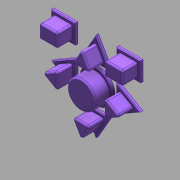
# Autodesk Inventor part: Button
Saved by Autodesk Inventor 2016 (Build 200138000, 138)
## iProperties
Created: 2016-08-15
Part Number: Button
Material: Water
Document SubType Name: Modeling
Designer: ADMIN
Density: 0.9983 g/cm^3
Appearance: Violet
Author: ADMIN
Autodesk Inventor part; units mm, degrees
ref_plane "YZ Plane" through (0, 0, 0) normal (1, 0, 0) x (0, 1, 0)
ref_plane "XZ Plane" through (0, 0, 0) normal (0, 1, 0) x (-1, 0, 0)
ref_plane "XY Plane" through (0, 0, 0) normal (0, 0, 1) x (1, 0, 0)
sketch "Sketch7" plane through (0, 0, 0) normal (0, 1, 0) x (-1, 0, 0)
  circle A0 centre (0, 0) radius 15
  line L0 (-25, 0) -> (-25, 10)
  line L1 (-25, 0) -> (-25, -10)
  line L2 (-25, -10) -> (-42.3205, 0)
  line L3 (-42.3205, 0) -> (-25, 10)
  line L4 (-22, 15.1962) -> (-22, 0)
  line L5 (-22, 0) -> (-22, -15.1962)
  line L6 (-22, -15.1962) -> (-48.3205, 0)
  line L7 (-48.3205, 0) -> (-22, 15.1962)
  circle A1 centre (0, 0) radius 18
  line L8 (0, -25) -> (-10, -25)
  line L9 (0, -25) -> (10, -25)
  line L10 (10, -25) -> (0, -42.3205)
  line L11 (0, -42.3205) -> (-10, -25)
  line L12 (-15.1962, -22) -> (0, -22)
  line L13 (0, -22) -> (15.1962, -22)
  line L14 (15.1962, -22) -> (0, -48.3205)
  line L15 (0, -48.3205) -> (-15.1962, -22)
  line L16 (25, 0) -> (25, -10)
  line L17 (25, 0) -> (25, 10)
  line L18 (25, 10) -> (42.3205, 0)
  line L19 (42.3205, 0) -> (25, -10)
  line L20 (22, -15.1962) -> (22, 0)
  line L21 (22, 0) -> (22, 15.1962)
  line L22 (22, 15.1962) -> (48.3205, 0)
  line L23 (48.3205, 0) -> (22, -15.1962)
  line L24 (0, 25) -> (10, 25)
  line L25 (0, 25) -> (-10, 25)
  line L26 (-10, 25) -> (0, 42.3205)
  line L27 (0, 42.3205) -> (10, 25)
  line L28 (15.1962, 22) -> (0, 22)
  line L29 (0, 22) -> (-15.1962, 22)
  line L30 (-15.1962, 22) -> (0, 48.3205)
  line L31 (0, 48.3205) -> (15.1962, 22)
  line L32 (48.3205, 48.3205) -> (22.3205, 48.3205)
  line L33 (22.3205, 48.3205) -> (22.3205, 27.3205)
  line L34 (22.3205, 27.3205) -> (48.3205, 27.3205)
  line L35 (48.3205, 27.3205) -> (48.3205, 48.3205)
  line L36 (-48.3205, 48.3205) -> (-22.3205, 48.3205)
  line L37 (-22.3205, 48.3205) -> (-22.3205, 27.3205)
  line L38 (-22.3205, 27.3205) -> (-48.3205, 27.3205)
  line L39 (-48.3205, 27.3205) -> (-48.3205, 48.3205)
  line L40 (45.3205, 45.3205) -> (25.3205, 45.3205)
  line L41 (25.3205, 45.3205) -> (25.3205, 30.3205)
  line L42 (25.3205, 30.3205) -> (45.3205, 30.3205)
  line L43 (45.3205, 30.3205) -> (45.3205, 45.3205)
  line L44 (-25.3205, 30.3205) -> (-25.3205, 45.3205)
  line L45 (-25.3205, 45.3205) -> (-45.3205, 45.3205)
  line L46 (-45.3205, 45.3205) -> (-45.3205, 30.3205)
  line L47 (-45.3205, 30.3205) -> (-25.3205, 30.3205)
  dimension "d85" = 10
  dimension "d86" = 10
  dimension "d87" = 20
  dimension "d88" = 60
  dimension "d89" = 3
  dimension "d90" = 3
  dimension "d93" = 360
  dimension "d95" = 26
  dimension "d96" = 21
  dimension "d97" = 26
  dimension "d98" = 21
  dimension "d99" = 3
  dimension "d100" = 3
  constraints: 96 end point, 8 parallel, 4 perpendicular, 2 centre point, 2 horizontal, 2 vertical, 1 coincident, 1 point on line, 74 other
  measures "d85" distance of L0.start L0.end
  measures "d86" distance of L0.start L1.end
  measures "d87" distance of L1.end L2.end
  measures "d88" angle of L1 L2
  measures "d89" distance between parallel lines of L0 L4
  measures "d90" radial gap between concentric circles of A0 A1
  measures "d95" distance of L34.end L33.end
  measures "d96" distance of L33.end L32.end
  measures "d97" distance of L37.end L38.end
  measures "d98" distance of L36.end L37.end
  measures "d99" distance between parallel lines of L35 L43
  measures "d100" distance between parallel lines of L37 L44
extrude "Extrusion3" add sketch "Sketch7" against normal blind 4
sketch "Sketch8" plane through (0, 0, 0) normal (0, 1, 0) x (1, 0, 0)
  line L0 (-25, -10) -> (-25, 10) projected
  line L1 (-25, -10) -> (-42.3205, 0) projected
  line L2 (-25, 10) -> (-42.3205, 0)
  line L3 (-42.3205, 0) -> (-25, -10)
  line L4 (-25, -10) -> (-25, 10)
  line L5 (-25.3205, -30.3205) -> (-45.3205, -30.3205) projected
  line L6 (-45.3205, -30.3205) -> (-25.3205, -30.3205)
  line L7 (-25.3205, -30.3205) -> (-25.3205, -45.3205)
  line L8 (-25.3205, -45.3205) -> (-45.3205, -45.3205)
  line L9 (-45.3205, -45.3205) -> (-45.3205, -30.3205)
  line L10 (25.3205, -30.3205) -> (45.3205, -30.3205)
  line L11 (45.3205, -30.3205) -> (45.3205, -45.3205)
  line L12 (45.3205, -45.3205) -> (25.3205, -45.3205)
  line L13 (25.3205, -45.3205) -> (25.3205, -30.3205)
  line L14 (-10, -25) -> (0, -42.3205)
  line L15 (0, -42.3205) -> (10, -25)
  line L16 (10, -25) -> (-10, -25)
  line L17 (25, -10) -> (42.3205, 0)
  line L18 (42.3205, 0) -> (25, 10)
  line L19 (25, 10) -> (25, -10)
  line L20 (10, 25) -> (0, 42.3205)
  line L21 (0, 42.3205) -> (-10, 25)
  line L22 (-10, 25) -> (10, 25)
  circle A0 centre (0, 0) radius 15
  dimension "d103" = 20
  dimension "d104" = 15
  dimension "d105" = 20
  dimension "d106" = 15
  dimension "d109" = 360
  dimension "d111" = 30
  constraints: 40 end point, 6 equal length, 2 horizontal, 2 perpendicular, 1 centre point, 1 coincident, 25 other
  measures "d103" distance of L7.end L8.end
  measures "d104" distance of L6.end L7.end
  measures "d105" distance of L11.end L12.end
  measures "d106" distance of L10.end L11.end
  measures "d111" diameter of A0
extrude "Extrusion4" add sketch "Sketch8" against normal blind 20
sketch "Sketch9" plane through (0, 0, 0) normal (0, 1, 0) x (1, 0, 0)
  circle A0 centre (-7.5, 0) radius 1.5
  circle A1 centre (0, -37) radius 1.5
  circle A2 centre (-40, -37.8205) radius 1.5
  circle A3 centre (40, -37.8205) radius 1.5
  circle A4 centre (37, 0) radius 1.5
  circle A5 centre (0, 37) radius 1.5
  circle A6 centre (-37, 0) radius 1.5
  point P0 (0, 0)
  dimension "d114" = 3
  dimension "d115" = 3
  dimension "d116" = 3
  dimension "d117" = 3
  dimension "d120" = 360
  constraints: 7 centre point, 9 other
  measures "d114" diameter of A0
  measures "d115" diameter of A1
  measures "d116" diameter of A2
  measures "d117" diameter of A3
extrude "Extrusion5" cut sketch "Sketch9" against normal blind 12
fillet "Fillet12" radius 2 21 edges at (45.3205, -12, 45.3205) (25.3205, -12, 45.3205) (25.3205, -12, 30.3205) (45.3205, -12, 30.3205) (42.3205, -12, 0) (25, -12, 10) (25, -12, -10) (0, -12, -42.3205) (-10, -12, -25) (10, -12, -25) (-42.3205, -12, 0) (-25, -12, -10) (-25, -12, 10) (-45.3205, -12, 30.3205) (-10, -12, 25) (0, -12, 42.3205) (-45.3205, -12, 45.3205) (-25.3205, -12, 45.3205) (10, -12, 25) (-25.3205, -12, 30.3205) (-15, -20, 0)
fillet "Fillet13" radius 2 40 edges at (44.7347, -20, 44.7347) (35.3205, -20, 45.3205) (25.9063, -20, 44.7347) (25.3205, -20, 37.8205) (25.9063, -20, 30.9063) (35.3205, -20, 30.3205) (44.7347, -20, 30.9063) (45.3205, -20, 37.8205) (0, -20, 40.3205) (-5, -20, 33.6603) (-8.2679, -20, 26) (0, -20, 25) (8.2679, -20, 26) (5, -20, 33.6603) (26, -20, 8.2679) (25, -20, 0) (26, -20, -8.2679) (33.6603, -20, -5) (40.3205, -20, 0) (33.6603, -20, 5) (-25.9063, -20, 44.7347) (-35.3205, -20, 45.3205) (-44.7347, -20, 44.7347) (-45.3205, -20, 37.8205) (-44.7347, -20, 30.9063) (-35.3205, -20, 30.3205) (-25.9063, -20, 30.9063) (-25.3205, -20, 37.8205) (-26, -20, 8.2679) (-33.6603, -20, 5) (-40.3205, -20, 0) (-33.6603, -20, -5) (-26, -20, -8.2679) (-25, -20, 0) (-8.2679, -20, -26) (-5, -20, -33.6603) (0, -20, -40.3205) (5, -20, -33.6603) (8.2679, -20, -26) (0, -20, -25)
fillet "Fillet14" radius 1 21 edges at (-35.3205, -4, 27.3205) (-48.3205, -4, 37.8205) (-35.3205, -4, 48.3205) (-22.3205, -4, 37.8205) (-7.5981, -4, 35.1603) (7.5981, -4, 22) (7.5981, -4, 35.1603) (22.3205, -4, 37.8205) (35.3205, -4, 27.3205) (48.3205, -4, 37.8205) (35.3205, -4, 48.3205) (-35.1603, -4, 7.5981) (-35.1603, -4, -7.5981) (-22, -4, 7.5981) (-7.5981, -4, -22) (-7.5981, -4, -35.1603) (7.5981, -4, -35.1603) (35.1603, -4, -7.5981) (22, -4, -7.5981) (35.1603, -4, 7.5981) (18, -4, 0)
fillet "Fillet15" radius 1 7 edges at (38.5, 0, 37.8205) (-1.5, 0, 37) (-41.5, 0, 37.8205) (-38.5, 0, 0) (-9, 0, 0) (35.5, 0, 0) (-1.5, 0, -37)
fillet "Fillet16" radius 1 21 edges at (18, 0, 0) (22, 0, 7.5981) (35.1603, 0, 7.5981) (35.1603, 0, -7.5981) (35.3205, 0, 27.3205) (22.3205, 0, 37.8205) (48.3205, 0, 37.8205) (35.3205, 0, 48.3205) (7.5981, 0, 35.1603) (-7.5981, 0, 22) (-7.5981, 0, 35.1603) (-22.3205, 0, 37.8205) (-35.3205, 0, 27.3205) (-48.3205, 0, 37.8205) (-35.3205, 0, 48.3205) (-35.1603, 0, 7.5981) (-22, 0, -7.5981) (-35.1603, 0, -7.5981) (-7.5981, 0, -35.1603) (7.5981, 0, -22) (7.5981, 0, -35.1603)
body "Solid2"
